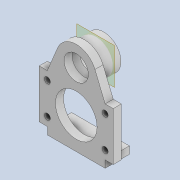
# Autodesk Inventor part: pin_conn_1
Saved by Autodesk Inventor 2020 (Build 240168000, 168)
## iProperties
Created: 2021-07-15
Part Number: pin_conn_1
Material: Generic
Document SubType Name: Modeling
Designer: Shuang Peng
Density: 1 g/cm^3
Appearance: Default
Author: Shuang Peng
Autodesk Inventor part; units mm, degrees
ref_plane "YZ Plane" through (0, 0, 0) normal (1, 0, 0) x (0, 1, 0)
ref_plane "XZ Plane" through (0, 0, 0) normal (0, 1, 0) x (-1, 0, 0)
ref_plane "XY Plane" through (0, 0, 0) normal (0, 0, 1) x (1, 0, 0)
sketch "Sketch1" plane through (0, 0, 0) normal (0, 0, 1) x (1, 0, 0)
  circle A0 centre (-7, 0) radius 1.5 projected
  circle A1 centre (7.15, -3.9) radius 0.75 projected
  circle A2 centre (-7.15, 3.9) radius 0.75 projected
  circle A3 centre (7.15, 3.9) radius 0.75 projected
  circle A4 centre (-7.15, -3.9) radius 0.75 projected
  circle A5 centre (0, 0) radius 3.5 projected
  arc A6 (-8.1536, -5.7895) -> (-7.746, -6) centre (-7.746, -5.5) ccw projected
  line L0 (7.746, -6) -> (-7.746, -6) projected
  arc A7 (7.746, -6) -> (8.1536, -5.7895) centre (7.746, -5.5) ccw projected
  arc A8 (8.1536, -5.7895) -> (8.1536, 5.7895) centre (0, 0) ccw projected
  arc A9 (8.1536, 5.7895) -> (7.746, 6) centre (7.746, 5.5) ccw projected
  line L1 (-7.746, 6) -> (7.746, 6) projected
  arc A10 (-7.746, 6) -> (-8.1536, 5.7895) centre (-7.746, 5.5) ccw projected
  arc A11 (-8.1536, 5.7895) -> (-8.1536, -5.7895) centre (0, 0) ccw projected
  line L2 (7.15, -3.9) -> (7.15, 3.9)
  line L3 (-7.15, -3.9) -> (-7.15, 3.9)
  line L4 (9.15, -6) -> (5.15, -6)
  line L5 (5.15, -6) -> (5.15, 6)
  line L6 (5.15, 6) -> (9.15, 6)
  line L7 (9.15, 6) -> (9.15, -6)
  line L8 (9.15, -6) -> (5.15, 6) construction
  line L9 (5.15, -6) -> (9.15, 6) construction
  line L10 (-5.15, -6) -> (-9.15, -6)
  line L11 (-9.15, -6) -> (-9.15, 6)
  line L12 (-9.15, 6) -> (-5.15, 6)
  line L13 (-5.15, 6) -> (-5.15, -6)
  line L14 (-5.15, -6) -> (-9.15, 6) construction
  line L15 (-9.15, -6) -> (-5.15, 6) construction
  circle A12 centre (0, 0) radius 8 projected
  circle A13 centre (0, 0) radius 8
  line L16 (0, 0) -> (0, 8)
  line L17 (0, 8) -> (0, 10.2)
  circle A14 centre (0, 10.2) radius 3
  circle A15 centre (0, 10.2) radius 5
  line L18 (7.15, 6) -> (4.6198, 12.1123)
  line L19 (-7.15, 6) -> (-4.6198, 12.1123)
  circle A16 centre (0, 0) radius 5.15
  point P0 (0, 0)
  point P1 (7.15, 0)
  point P2 (-7.15, 0)
  point P3 (-5.15, 0)
  point P4 (5.15, 0)
  dimension "d4" = 16
  dimension "d0" = 4
  dimension "d1" = 12
  dimension "d2" = 4
  dimension "d3" = 12
  dimension "d5" = 2.2
  dimension "d6" = 6
  dimension "d7" = 10
  constraints: 36 end point, 9 midpoint, 4 coincident, 4 parallel, 4 perpendicular, 4 vertical, 2 centre point, 2 point on circle, 2 tangent, 1 vertical alignment, 5 other
  measures "d0" distance of L4.start L4.end
  measures "d1" distance of L4.end L5.end
  measures "d2" distance of L10.start L10.end
  measures "d3" distance of L10.end L11.end
  measures "d5" distance of L16.end L17.end
  measures "d6" diameter of A14
  measures "d7" diameter of A15
extrude "Extrusion1" add sketch "Sketch1" along normal blind 2 contours A0 L3 | A0 L3 A2 A12 L1 L13 L0 A4 | L3 A0 A12 | A0 A12 A2 L3 | L3 A4 A12 A0 | A12 A0 | A0 A12 A4 L0 A6 A11 L11 A10 L1 A2 | A12 A15 L1 | L1 L19 A15 A12 | L1 A15 L16 A16 L13 | A15 A12 A14 | A12 A14 L16 L1 A15 | L10 L11 A11 A6 | A12 A1 A3 L1 A9 A8 L7 A7 L0 | L0 L5 L1 A12 A3 L2 A1 | A10 A11 L11 L12 | L1 L16 A15 | A7 A8 L7 L4 | L18 L1 A12 A15 | L16 A14 A12 A15 L1 | L1 A15 L16 | A15 L1 L5 A16 L16 | L2 A3 A12 A1 | A15 A12 L1 | L6 L7 A8 A9
sketch "Sketch2" plane through (0, 0, 0) normal (0, 0, -1) x (-1, 0, 0)
  line L0 (-5.15, 0) -> (-5.15, -6) projected
  arc A0 (5.15, 0) -> (-5.15, 0) centre (0, 0) ccw projected
  line L1 (5.15, -6) -> (5.15, 0) projected
  line L2 (9.15, -6) -> (5.15, -6) projected
  line L3 (9.15, 6) -> (9.15, -6) projected
  line L4 (7.15, 6) -> (9.15, 6) projected
  line L5 (4.6198, 12.1123) -> (7.15, 6) projected
  arc A1 (4.6198, 12.1123) -> (-4.6198, 12.1123) centre (0, 10.2) ccw projected
  line L6 (-7.15, 6) -> (-4.6198, 12.1123) projected
  line L7 (-9.15, 6) -> (-7.15, 6) projected
  line L8 (-9.15, -6) -> (-9.15, 6) projected
  line L9 (-5.15, -6) -> (-9.15, -6) projected
  circle A2 centre (-7.15, 3.9) radius 0.75 projected
  circle A3 centre (7.15, -3.9) radius 0.75 projected
  circle A4 centre (7.15, 3.9) radius 0.75 projected
  circle A5 centre (-7.15, -3.9) radius 0.75 projected
  circle A6 centre (0, 10.2) radius 3 projected
  circle A7 centre (0, 10.2) radius 3 projected
  circle A8 centre (0, 10.2) radius 4.25
  point P0 (0, 0)
  dimension "d10" = 8.5
  constraints: 1 centre point, 1 coincident
  measures "d10" diameter of A8
extrude "Extrusion2" add sketch "Sketch2" along normal blind 4.8 contours A8
sketch "Sketch3" plane through (0, 10.2, -4.8) normal (0, 0, -1) x (-1, 0, 0)
  circle A0 centre (0, 0) radius 4.25 projected
  circle A1 centre (0, 0) radius 3 projected
  line L0 (0, 0) -> (4.25, 0)
  line L1 (0, 0) -> (0, -3.9)
  line L2 (0, -3.9) -> (1.6889, -3.9)
  line L3 (0, -3.9) -> (-1.6889, -3.9)
  circle A2 centre (0, 0) radius 4.25 projected
  point P0 (0, -10.2)
  dimension "d13" = 3.9
  constraints: 8 end point, 3 horizontal, 3 point on circle, 1 perpendicular
  measures "d13" distance of L0.start L1.end
extrude "Extrusion3" cut sketch "Sketch3" against normal up to surface (4.8 mm away) contours L3 L2 A0
ref_plane "Work Plane1" through (0, 0, -2.8) normal (0, 0, -1) x (-1, 0, 0)
sketch "Sketch4" plane through (0, 0, -2.8) normal (0, 0, -1) x (-1, 0, 0)
  circle A0 centre (0, 10.2) radius 3 projected
  circle A1 centre (0, 10.2) radius 2
  point P0 (0, 0)
  dimension "d17" = 1
  constraints: 1 centre point, 1 coincident
  measures "d17" radial gap between concentric circles of A0 A1
extrude "Extrusion4" add sketch "Sketch4" against normal blind 2.8
chamfer "Chamfer1" distance 1 angle 45 2 edges at (2, 10.2, 0) (2, 10.2, -2.8)
sketch "Sketch5" plane through (0, 0, 0) normal (0, 0, -1) x (-1, 0, 0)
  arc A0 (1.6889, 6.3) -> (-1.6889, 6.3) centre (0, 10.2) ccw projected
  line L0 (1.6889, 6.3) -> (-1.6889, 6.3) projected
  line L1 (-5.15, 0) -> (-5.15, -6) projected
  arc A1 (5.15, 0) -> (-5.15, 0) centre (0, 0) ccw projected
  line L2 (5.15, -6) -> (5.15, 0) projected
  line L3 (9.15, -6) -> (5.15, -6) projected
  line L4 (9.15, 6) -> (9.15, -6) projected
  line L5 (7.15, 6) -> (9.15, 6) projected
  line L6 (4.6198, 12.1123) -> (7.15, 6) projected
  arc A2 (4.6198, 12.1123) -> (-4.6198, 12.1123) centre (0, 10.2) ccw projected
  line L7 (-7.15, 6) -> (-4.6198, 12.1123) projected
  line L8 (-9.15, 6) -> (-7.15, 6) projected
  line L9 (-9.15, -6) -> (-9.15, 6) projected
  line L10 (-5.15, -6) -> (-9.15, -6) projected
  circle A3 centre (-7.15, 3.9) radius 0.75 projected
  circle A4 centre (7.15, -3.9) radius 0.75 projected
  circle A5 centre (7.15, 3.9) radius 0.75 projected
  circle A6 centre (-7.15, -3.9) radius 0.75 projected
  circle A7 centre (0, 0) radius 5.15
  line L11 (0, 0) -> (0, -5.15)
  line L12 (9.15, -6) -> (5.15, -6) projected
  line L13 (-5.15, 0) -> (-5.15, -6) projected
  line L14 (5.15, -6) -> (-5.15, -6)
  line L15 (-5.15, -6) -> (-9.15, -6) projected
  line L16 (-7.15, -6) -> (7.15, -6)
  line L17 (7.15, -6) -> (7.15, -7.8)
  line L18 (7.15, -7.8) -> (-7.15, -7.8)
  line L19 (-7.15, -7.8) -> (-7.15, -6)
  point P0 (0, 0)
  dimension "d23" = 10.3
  dimension "d24" = 14.3
  dimension "d25" = 1.8
  constraints: 12 end point, 2 parallel, 2 perpendicular, 1 coincident, 1 horizontal, 1 midpoint, 1 vertical, 3 other
  measures "d24" distance of L17.end L18.end
  measures "d25" distance of L16.end L17.end
extrude "Extrusion5" add sketch "Sketch5" against normal up to surface (2 mm away) contours A7 L2 L14 L1 | L14 L3 L17 L18 L19 L10
sketch "Sketch6" plane through (0, 0, 0) normal (0, 0, -1) x (-1, 0, 0)
  line L0 (9.15, -6) -> (7.15, -6) projected
  line L1 (9.15, 6) -> (9.15, -6) projected
  line L2 (7.15, 6) -> (9.15, 6) projected
  line L3 (4.6198, 12.1123) -> (7.15, 6) projected
  arc A0 (4.6198, 12.1123) -> (-4.6198, 12.1123) centre (0, 10.2) ccw projected
  line L4 (-7.15, 6) -> (-4.6198, 12.1123) projected
  line L5 (-9.15, 6) -> (-7.15, 6) projected
  line L6 (-9.15, -6) -> (-9.15, 6) projected
  line L7 (-7.15, -6) -> (-9.15, -6) projected
  line L8 (-7.15, -6) -> (-7.15, -7.8) projected
  line L9 (-7.15, -7.8) -> (7.15, -7.8) projected
  line L10 (7.15, -7.8) -> (7.15, -6) projected
  arc A1 (1.6889, 6.3) -> (-1.6889, 6.3) centre (0, 10.2) ccw projected
  line L11 (1.6889, 6.3) -> (-1.6889, 6.3) projected
  circle A2 centre (0, 0) radius 5.15 projected
  circle A3 centre (-7.15, 3.9) radius 0.75 projected
  circle A4 centre (7.15, -3.9) radius 0.75 projected
  circle A5 centre (7.15, 3.9) radius 0.75 projected
  circle A6 centre (-7.15, -3.9) radius 0.75 projected
  line L12 (-7.15, -7.8) -> (7.15, -7.8) projected
  line L13 (9.15, -6) -> (7.15, -6) projected
  line L14 (-7.15, -7.8) -> (7.15, -7.8)
  line L15 (7.15, -7.8) -> (7.15, -6)
  line L16 (7.15, -6) -> (-7.15, -6)
  line L17 (-7.15, -6) -> (-7.15, -7.8)
  point P0 (0, 0)
  constraints: 8 end point, 2 parallel, 1 horizontal, 1 perpendicular
extrude "Extrusion6" add sketch "Sketch6" along normal blind 4 contours L10 L9 L8 L16
body "Solid1"
